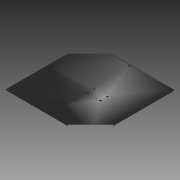
# Autodesk Inventor part: EnclosurePanelLeft
Saved by Autodesk Inventor 2016 (Build 200138000, 138)
## iProperties
Category: Panel
Created: 2015-01-12
Part Number: EnclosurePanelLeft
Material: ABS Plastic
Document SubType Name: Modeling
Designer: Jack
Density: 1.06 g/cm^3
Appearance: Smooth - Dark Gray
Mass: 876.625 g
Surface Area: 3566.9 cm^2
Volume: 827.005 cm^3
Vendor: Tap Plastics
Catalog Web Link: N/A
Author: Jack
Title: Enclosure Panel Left
Autodesk Inventor part; units mm, degrees
ref_plane "YZ Plane" through (0, 0, 0) normal (1, 0, 0) x (0, 1, 0)
ref_plane "XZ Plane" through (0, 0, 0) normal (0, 1, 0) x (-1, 0, 0)
ref_plane "XY Plane" through (0, 0, 0) normal (0, 0, 1) x (1, 0, 0)
sketch "Sketch1" plane through (0, 0, 0) normal (0, 0, 1) x (1, 0, 0)
  line L0 (0, 0) -> (424.7625, 0)
  line L1 (424.7625, 0) -> (424.7625, 420)
  line L2 (424.7625, 420) -> (0, 420)
  line L3 (0, 420) -> (0, 0)
  dimension "d0" = 424.7625
  dimension "d1" = 420
  constraints: 8 end point, 2 parallel, 1 horizontal, 1 perpendicular
  measures "d0" distance of L2.end L1.end
  measures "d1" distance of L0.end L1.end
extrude "Extrusion1" add sketch "Sketch1" along normal blind 4.7625
sketch "Sketch6" plane through (0, 0, 4.7625) normal (0, 0, 1) x (1, 0, 0)
  line L0 (0, 0) -> (424.7625, 0) projected
  line L1 (424.7625, 0) -> (424.7625, 420) projected
  line L2 (424.7625, 420) -> (0, 420) projected
  line L3 (0, 420) -> (0, 0) projected
  circle A0 centre (14.7625, 410) radius 2.25
  circle A1 centre (414.7625, 410) radius 2.25
  circle A2 centre (14.7625, 10) radius 2.25
  circle A3 centre (414.7625, 10) radius 2.25
  circle A4 centre (14.7625, 210) radius 2.25
  circle A5 centre (414.7625, 210) radius 2.25
  circle A6 centre (209.8815, 410) radius 2.25
  circle A7 centre (209.8815, 10) radius 2.25
  circle A8 centre (209.8815, 75) radius 2.25
  dimension "d42" = 4.5
  dimension "d43" = 10
  dimension "d44" = 14.7625
  dimension "d45" = 10
  dimension "d46" = 10
  dimension "d47" = 10
  dimension "d48" = 210
  dimension "d51" = 209.8815
  dimension "d55" = 75
  constraints: 9 centre point, 8 equal radius, 6 vertical alignment, 4 horizontal alignment
  measures "d42" diameter of A0
  measures "d43" distance from line of L2 A0.centre
  measures "d44" distance from line of L3 A0.centre
  measures "d45" distance from line of L1 A1.centre
  measures "d46" distance from line of L2 A1.centre
  measures "d47" distance from line of L0 A2.centre
  measures "d48" distance from line of L0 A5.centre
  measures "d51" distance from line of L3 A6.centre
  measures "d55" distance from line of L0 A8.centre
extrude "Extrusion3" cut sketch "Sketch6" against normal up to next contours A0 | A1 | A2 | A3 | A4 | A5 | A6 | A7 | A8
chamfer "Chamfer1" distance 2 angle 45 9 edges at (12.5125, 410, 4.7625) (207.6315, 410, 4.7625) (412.5125, 410, 4.7625) (412.5125, 210, 4.7625) (12.5125, 210, 4.7625) (12.5125, 10, 4.7625) (207.6315, 10, 4.7625) (412.5125, 10, 4.7625) (207.6315, 75, 4.7625)
sketch "Sketch7" plane through (0, 0, 4.7625) normal (0, 0, 1) x (1, 0, 0)
  line L0 (0, 0) -> (424.7625, 0) projected
  line L1 (424.7625, 0) -> (424.7625, 420) projected
  line L2 (424.7625, 420) -> (0, 420) projected
  line L3 (0, 420) -> (0, 0) projected
  line L4 (424.7625, 180) -> (0, 180) construction
  line L5 (424.7625, 420) -> (0, 420) construction
  line L6 (294.7625, 420) -> (294.7625, 0) construction
  point P0 (222.2625, 222.5)
  point P1 (287.2625, 222.5)
  point P2 (222.2625, 187.5)
  point P3 (287.2625, 187.5)
  dimension "d56" = 180
  dimension "d57" = 130
  dimension "d58" = 7.5
  dimension "d59" = 7.5
  dimension "d60" = 65
  dimension "d61" = 35
  constraints: 4 end point, 4 point on line, 2 horizontal alignment, 2 perpendicular, 2 vertical alignment
  measures "d56" distance between parallel lines of L0 L4
  measures "d57" distance between parallel lines of L1 L6
  measures "d58" distance from line of L6 point (287.262, 187.5)
  measures "d59" distance from line of L4 point (287.262, 187.5)
  measures "d60" distance of point (222.262, 187.5) point (287.262, 187.5)
  measures "d61" distance of point (287.262, 187.5) point (287.262, 222.5)
hole "Hole3" at (222.2625, 222.5, 4.7625) at (287.2625, 222.5, 4.7625) at (222.2625, 187.5, 4.7625) at (287.2625, 187.5, 4.7625) direction (0, 0, -1) diameter 4.5 end through all countersink diameter 8.5 countersink angle 90
body "Solid1"
